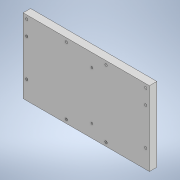
# Autodesk Inventor part: base
Saved by Autodesk Inventor 2022.2 (Build 262287030, 287C)
## iProperties
Created: 2022-01-28
Part Number: base
Material: Generic
Document SubType Name: Modeling
Designer: Tapendra
Density: 1 g/cm^3
Appearance: Default
Author: Tapendra
Autodesk Inventor part; units mm, degrees
ref_plane "YZ Plane" through (0, 0, 0) normal (1, 0, 0) x (0, 1, 0)
ref_plane "XZ Plane" through (0, 0, 0) normal (0, 1, 0) x (-1, 0, 0)
ref_plane "XY Plane" through (0, 0, 0) normal (0, 0, 1) x (1, 0, 0)
sketch "Sketch1" plane through (0, 0, 0) normal (0, 0, 1) x (1, 0, 0)
  line L0 (-85, 50) -> (85, 50)
  line L1 (85, 50) -> (85, -50)
  line L2 (85, -50) -> (-85, -50)
  line L3 (-85, -50) -> (-85, 50)
  line L4 (-85, 50) -> (85, -50) construction
  line L5 (85, 50) -> (-85, -50) construction
  point P0 (0, 0)
  dimension "d0" = 170
  dimension "d1" = 100
  constraints: 12 end point, 2 midpoint, 2 parallel, 1 horizontal, 1 perpendicular
  measures "d0" distance of L0.start L0.end
  measures "d1" distance of L0.end L1.end
extrude "Extrusion1" add sketch "Sketch1" along normal mid plane 10
sketch "Sketch2" plane through (0, 0, 5) normal (0, 0, 1) x (1, 0, 0)
  line L0 (-85, 50) -> (-85, -50) projected
  line L1 (-85, -50) -> (85, -50) projected
  line L2 (85, -50) -> (85, 50) projected
  line L3 (85, 50) -> (-85, 50) projected
  line L4 (-85, 50) -> (-85, -50) projected
  point P0 (0, 0)
  point P1 (80, 45)
  point P2 (26.6667, 45)
  point P3 (-80, 45)
  point P4 (80, 25)
  point P5 (80, -25)
  point P6 (-80, 25)
  point P7 (-80, -25)
  point P8 (-26.6667, 45)
  point P9 (26.6667, -45)
  point P10 (-26.6667, -45)
  dimension "d17" = 53.3333
  dimension "d53" = 50
  dimension "d61" = 160
  dimension "d68" = 160
  dimension "d73" = 5
  dimension "d74" = 5
  dimension "d75" = 5
  dimension "d77" = 5
  dimension "d112" = 53.3333
  dimension "d115" = 90
  dimension "d118" = 25
  constraints: 3 horizontal, 2 vertical, 6 other
  measures "d17" distance of point (80, 45) point (26.667, 45)
  measures "d53" distance of point (80, 25) point (80, -25)
  measures "d61" distance of point (80, 25) point (-80, 25)
  measures "d68" distance of point (80, -25) point (-80, -25)
  measures "d73" distance from line of L0 point (-80, 45)
  measures "d74" distance from line of L2 point (80, 45)
  measures "d75" distance from line of L3 point (80, 45)
  measures "d77" distance from line of L3 point (-80, 45)
  measures "d112" distance of point (26.667, 45) point (-26.667, 45)
  measures "d115" distance of point (26.667, 45) point (26.667, -45)
  measures "d118" vertical distance of point (80, 25) point (0, 0)
hole "Hole1" at (-80, 45, 5) at (26.6667, 45, 5) at (80, 45, 5) at (80, 25, 5) at (80, -25, 5) at (-80, 25, 5) at (-80, -25, 5) at (-26.6667, 45, 5) at (-26.6667, -45, 5) at (26.6667, -45, 5) direction (0, 0, -1) diameter 3.175 depth 5
sketch "Sketch3" plane through (0, 0, -5) normal (0, 0, -1) x (-1, 0, 0)
  point P0 (0, 0)
  point P1 (0, 15)
  point P2 (-15, 0)
  point P3 (0, -15)
  point P4 (15, 0)
  dimension "d81" = 15
  dimension "d84" = 360
  constraints: 1 vertical alignment, 5 other
  measures "d81" distance of point (0, 15) point (0, 0)
hole "Hole2" at (0, 15, -5) at (15, 0, -5) at (0, -15, -5) at (-15, 0, -5) direction (0, 0, 1) diameter 2.5 depth 3
sketch "Sketch4" plane through (0, 0, 5) normal (0, 0, 1) x (1, 0, 0)
  line L0 (85, -50) -> (85, 50) projected
  line L1 (-85, 50) -> (-85, -50) projected
  point P0 (0, 0)
  point P1 (7.62, 32.5)
  point P2 (7.62, -32.5)
  dimension "d94" = 32.5
  dimension "d97" = 65
  dimension "d109" = 92.62
  constraints: 1 vertical, 1 other
  measures "d94" vertical distance of point (7.62, 32.5) point (0, 0)
  measures "d97" distance of point (7.62, 32.5) point (7.62, -32.5)
  measures "d109" distance from line of L1 point (7.62, 32.5)
hole "Hole3" at (7.62, 32.5, 5) at (7.62, -32.5, 5) direction (0, 0, -1) diameter 2.5 depth 3
equation "\"d17\" = 0.333333 * d61"
equation "\"d112\" = d17"
equation "\"d118\" = 0.5 * d53"
body "Solid1"
